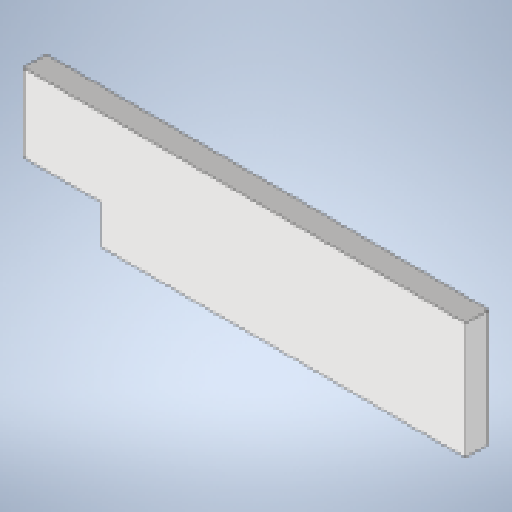
# Autodesk Inventor part: ДМФ 094 Постель НОС крепление v2.0
Saved by Autodesk Inventor 2025 (Build 290162010, 162A)
## iProperties
Created: 2024-04-28
Part Number: ДМФ 094 Постель НОС крепление v2.0
Material: Generic
Document SubType Name: Sheet Metal
Designer: pokla
Stock Number: Постель_Нос
Density: 1 g/cm^3
Sheet Metal Rule: Default
Sheet Metal Width: 0,000 mm
Sheet Metal Length: 0,000 mm
Sheet Metal Area: 0,000 mm^2
Appearance: Default
Author: pokla
Autodesk Inventor part; units mm, degrees
ref_plane "YZ Plane" through (0, 0, 0) normal (1, 0, 0) x (0, 1, 0)
ref_plane "XZ Plane" through (0, 0, 0) normal (0, 1, 0) x (-1, 0, 0)
ref_plane "XY Plane" through (0, 0, 0) normal (0, 0, 1) x (1, 0, 0)
sketch "Sketch9" plane through (0, 0, 0) normal (0, 0, 1) x (1, 0, 0)
  line L0 (-60, 15) -> (60, 15)
  line L1 (60, 15) -> (60, -15)
  line L2 (60, -15) -> (-60, -15)
  line L3 (-60, -15) -> (-60, 15)
  line L4 (-60, 15) -> (60, -15) construction
  line L5 (-54, 15) -> (-54, -15)
  line L6 (-34, 15) -> (-34, -15)
  line L7 (-60, -5) -> (-34, -5)
  point P0 (0, 0)
  point P1 (0, 0)
  point P2 (-54, -5)
  dimension "d58" = 120
  dimension "d59" = 30
  dimension "d66" = 6
  dimension "d67" = 26
  dimension "d68" = 10
  measures "d58" distance of L0.start L0.end
  measures "d59" distance of L2.end L0.start
  measures "d66" distance between parallel lines of L5 L3
  measures "d67" distance between parallel lines of L6 L3
  measures "d68" distance between parallel lines of L2 L7
extrude "Plate2" add sketch "Sketch9" against normal blind 6 contours L0 L6 L7 L5 | L0 L1 L2 L6
sketch "Sketch11" plane through (0, 0, 0) normal (0, 0, 1) x (1, 0, 0)
  circle A0 centre (35, 0) radius 7
  line L0 (60, -15) -> (60, 15) projected
  point P0 (0, 0)
  dimension "d69" = 25
  dimension "d70" = 14
  constraints: 1 centre point, 1 horizontal alignment
  measures "d69" distance from line of L0 A0.centre
  measures "d70" diameter of A0
extrude "Cut1" cut sketch "Sketch11" against normal through all
equation "\"d71\" = Thickness"
equation "\"d60\" = Thickness"
equation "\"BendRadius\" = Thickness"
equation "\"BendReliefWidth\" = Thickness"
equation "\"BendReliefDepth\" = 0.5 * Thickness"
equation "\"CornerReliefSize\" = 4 * Thickness"
equation "\"MinimumRemnant\" = 2 * Thickness"
equation "\"TransitionRadius\" = BendRadius"
equation "\"JacobiRadiusSize\" = BendRadius"
equation "\"GapSize\" = Thickness"
equation "\"Thickness\" = 6"
body "Solid3"
